StratoSoar Rev2-f3d (Autodesk Fusion 360 design; units mm, degrees)
Autodesk Fusion 360 part; units mm, degrees
sketch "Sketch1" plane through (0, 0, 0) normal (0, 1, 0) x (1, 0, 0)
  circle A0 centre (0, 0) radius 1.5
  dimension "d1" = 3
  constraint coincident A0.centre origin
  measures "d1" diameter of A0
extrude "Extrude1" add sketch "Sketch1" along normal blind 500
extrude "Extrude2" add 1 faces at (0.567, 500, 0.5383) along direction (0, 1, 0) blind 5
extrude "Extrude3" add 1 faces at (0.567, 505, 0.5383) along direction (0, 1, 0) blind 4
